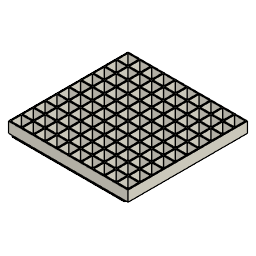
wortuhr (Autodesk Fusion 360 design; units mm, degrees)
Autodesk Fusion 360 part; units mm, degrees
sketch "Skizze1" plane through (0, 0, 0) normal (0, 0, 1) x (1, 0, 0)
  line L0 (83.75, 83.75) -> (-83.75, 83.75)
  line L1 (-83.75, 83.75) -> (-83.75, -83.75)
  line L2 (-83.75, -83.75) -> (83.75, -83.75)
  line L3 (83.75, -83.75) -> (83.75, 83.75)
  line L4 (83.75, 83.75) -> (-83.75, -83.75) construction
  line L5 (-83.75, 83.75) -> (83.75, -83.75) construction
  dimension "d7" = 167.5
  dimension "d8" = 167.5
  constraint horizontal L0
  constraint perpendicular L0 L1
  constraint parallel L0 L2
  constraint parallel L1 L3
  constraint coincident L4 origin
  constraint coincident L5 origin
  measures "d7" distance of L1.end L2.end
  measures "d8" distance of L0.end L1.end
extrude "Extrusion1" add sketch "Skizze1" along normal blind 15 makes body 1
sketch "Skizze2" plane through (0, 0, 15) normal (0, 0, 1) x (-1, 0, 0)
  line L0 (-83.75, 83.75) -> (-83.75, -83.75)
  line L1 (-83.75, -83.75) -> (83.75, -83.75)
  line L2 (83.75, -83.75) -> (83.75, 83.75)
  line L3 (83.75, 83.75) -> (-83.75, 83.75)
  line L4 (83.75, -83.75) -> (83.75, 83.75)
  line L5 (83.75, 83.75) -> (-83.75, 83.75)
  line L6 (82.25, 82.25) -> (67.15, 82.25)
  line L7 (67.15, 82.25) -> (67.15, 67.15)
  line L8 (67.15, 67.15) -> (82.25, 67.15)
  line L9 (82.25, 67.15) -> (82.25, 82.25)
  line L10 (79.2, 70.2) -> (70.2, 70.2)
  line L11 (70.2, 70.2) -> (70.2, 79.2)
  line L12 (70.2, 79.2) -> (79.2, 79.2)
  line L13 (79.2, 79.2) -> (79.2, 70.2)
  dimension "d12" = 15.1
  dimension "d13" = 15.1
  dimension "d14" = 1.5
  dimension "d15" = 1.5
  dimension "d16" = 3.05
  dimension "d18" = 9
  dimension "d19" = 9
  dimension "d20" = 3.05
  constraint horizontal L6
  constraint vertical L7
  constraint horizontal L8
  constraint vertical L9
  constraint horizontal L10
  constraint vertical L11
  constraint horizontal L12
  constraint vertical L13
  measures "d12" distance of L6.start L8.end
  measures "d13" distance of L7 L9
  measures "d14" distance of L4 L9
  measures "d15" distance of L5 L6
  measures "d16" distance of L9 L13
  measures "d18" distance of L11 L13
  measures "d19" distance of L10 L12
  measures "d20" distance of L6 L12
extrude "Extrusion2" cut sketch "Skizze2" against normal blind 15 contours L10 L11 L12 L13 bodies 1
extrude "Extrusion3" cut sketch "Skizze2" against normal blind 13.5 contours L6 L7 L8 L9 bodies 1
pattern_linear "R-Anordnung1" count 10 spacing 16.6 along (0, 1, 0) count 10 spacing 16.6 along (1, 0, 0) of "Extrusion2", "Extrusion3"
extrude "Extrusion4" add sketch "Skizze1" against normal blind 2 separate body makes body 2
sketch "Skizze5" plane through (0, 0, 0) normal (0, 0, 1) x (1, 0, 0)
  line L0 (-83.75, -83.75) -> (83.75, -83.75)
  line L1 (-83.75, 83.75) -> (-83.75, -83.75)
  line L2 (-83.75, -83.75) -> (-78.75, -83.75)
  line L3 (-78.75, -83.75) -> (-78.75, -64.15)
  line L4 (-78.75, -64.15) -> (-83.75, -64.15)
  line L5 (-83.75, -64.15) -> (-83.75, -83.75)
  line L6 (83.75, -83.75) -> (78.75, -83.75)
  line L7 (78.75, -83.75) -> (78.75, -64.15)
  line L8 (78.75, -64.15) -> (83.75, -64.15)
  line L9 (83.75, -64.15) -> (83.75, -83.75)
  line L10 (-78.75, -71.95) -> (78.75, -71.95)
  line L11 (78.75, -71.95) -> (78.75, -77.45)
  line L12 (78.75, -77.45) -> (-78.75, -77.45)
  line L13 (-78.75, -77.45) -> (-78.75, -71.95)
  dimension "d43" = 5
  dimension "d44" = 19.6
  dimension "d45" = 19.6
  dimension "d46" = 5
  dimension "d47" = 157.5
  dimension "d48" = 5.5
  dimension "d49" = 6.3
  constraint horizontal L2
  constraint vertical L3
  constraint horizontal L4
  constraint vertical L5
  constraint coincident L0.start L1.end
  constraint horizontal L6
  constraint vertical L7
  constraint horizontal L8
  constraint vertical L9
  constraint coincident L0.end L6.start
  constraint horizontal L10
  constraint vertical L11
  constraint horizontal L12
  constraint vertical L13
  constraint collinear L3 L13
  measures "d43" distance of L0.start L2.end
  measures "d44" distance of L0.start L4.end
  measures "d45" distance of L0.end L8.end
  measures "d46" distance of L7.end L8.end
  measures "d47" distance of L10.start L10.end
  measures "d48" distance of L10.start L12.end
  measures "d49" distance of L0 L12
extrude "Extrusion5" cut sketch "Skizze5" against normal blind 2 contours L0 L1 L2 L3 L4 L5 L13 bodies 2
extrude "Extrusion6" cut sketch "Skizze5" against normal blind 2 contours L0 L6 L7 L8 L9 L11 bodies 2
extrude "Extrusion7" cut sketch "Skizze5" against normal blind 0.4 contours L3 L7 L10 L11 L12 L13 bodies 2
pattern_linear "R-Anordnung2" count 10 spacing 16.6 along (0, 1, 0) of "Extrusion5", "Extrusion6", "Extrusion7"
equation "ledPitch = 16.6 mm" comment "Abstand der LEDs auf dem Stripe"
equation "gridWallThk = 1.5 mm" comment "Dicke der Gitterwände"
equation "rows = 10" comment "Anzahl der Reihen"
equation "cols = 10" comment "Anzahl der Spalten"
equation "gridXSize = ( cols * ledPitch ) + gridWallThk" comment "Breite des gesamten Gitters"
equation "gridYSize = ( rows * ledPitch ) + gridWallThk" comment "Höhe des gesamten Gitters"
equation "d7 = gridXSize"
equation "d8 = gridYSize"
equation "gridDepth = 15 mm" comment "Tiefe des Gritters"
equation "d10 = gridDepth"
equation "d12 = ledPitch - gridWallThk"
equation "d13 = ledPitch - gridWallThk"
equation "d14 = gridWallThk"
equation "d15 = gridWallThk"
equation "d16 = ( ledPitch - gridWallThk ) / 2 - ( ledCutoutSize / 2 )"
equation "ledCutoutSize = 9 mm" comment "Seitenlänge des Quadratischen Cutouts für die LEDs auf dem Bank"
equation "d18 = ledCutoutSize"
equation "d19 = ledCutoutSize"
equation "d20 = ( ledPitch - gridWallThk ) / 2 - ( ledCutoutSize / 2 )"
equation "d21 = -gridDepth"
equation "d23 = -gridDepth + gridWallThk"
equation "d25 = rows"
equation "d26 = cols"
equation "d27 = ledPitch"
equation "d28 = ledPitch"
equation "solderCutoutSize = 5 mm" comment "Ausschnitte für das Löten der LED-Strips"
equation "carrierPlateThk = 2 mm" comment "LED Trägerplatten dicke"
equation "d32 = -carrierPlateThk"
equation "ledStripeWidth = 5.5 mm" comment "Breite des LED Strips für die Kleberinne"
equation "ledStripeHeight = 0.4 mm" comment "Höhe des LED Strips für die Kleberinne"
equation "d43 = solderCutoutSize"
equation "d44 = ledPitch + gridWallThk * 2"
equation "d45 = ledPitch + gridWallThk * 2"
equation "d46 = solderCutoutSize"
equation "d47 = gridXSize - 2 * solderCutoutSize"
equation "d48 = ledStripeWidth"
equation "d49 = ledPitch / 2 - ledStripeWidth / 2 + gridWallThk / 2"
equation "d50 = -carrierPlateThk"
equation "d52 = -carrierPlateThk"
equation "d54 = -ledStripeHeight"
equation "d56 = rows"
equation "d58 = -ledPitch"
named bodies: "Gitter", "Trägerplatte"
